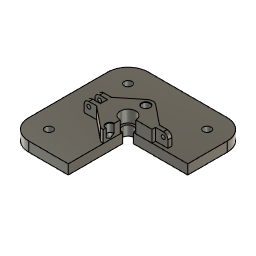
Sketch29_Final v2 (Autodesk Fusion 360 design; units mm, degrees)
Autodesk Fusion 360 part; units mm, degrees
sketch "Sketch2" plane through (0, 0, 0) normal (0, 0, 1) x (1, 0, 0)
  line L0 (102.0126, -154) -> (-102.0126, -154)
  line L1 (-154, -102.0126) -> (-154, 102.0126)
  line L2 (-102.0126, 154) -> (102.0126, 154)
  line L3 (154, 102.0126) -> (154, -102.0126)
  line L4 (138.7696, -138.7696) -> (-138.7696, 138.7696) construction
  line L5 (-138.7696, -138.7696) -> (138.7696, 138.7696) construction
  line L6 (0, 154) -> (-102, 154)
  line L7 (-154, 0) -> (-154, 102)
  circle A0 centre (-102, 102) radius 10
  circle A1 centre (102, 102) radius 10
  line L8 (-154, 0) -> (154, 0)
  circle A2 centre (-102, -102) radius 10
  circle A3 centre (102, -102) radius 10
  arc A4 (-101.9874, 154) -> (-154, 101.9874) centre (-102, 102) ccw
  arc A5 (154, 101.9874) -> (101.9874, 154) centre (102, 102) ccw
  arc A6 (101.9874, -154) -> (154, -101.9874) centre (102, -102) ccw
  arc A7 (-154, -101.9874) -> (-101.9874, -154) centre (-102, -102) ccw
  circle A8 centre (0, 0) radius 14
  dimension "d3" = 102
  dimension "d4" = 102
  dimension "d5" = 20
  dimension "d7" = 104
  dimension "d8" = 28
  constraint horizontal L0
  constraint perpendicular L0 L1
  constraint parallel L0 L2
  constraint parallel L1 L3
  constraint coincident L4 A8.centre
  constraint coincident L5 A8.centre
  constraint coincident A8.centre origin
  constraint parallel L2 L6
  constraint parallel L1 L7
  constraint coincident L4 A0.centre
  constraint concentric A0 A4
  constraint coincident L1.end A4
  constraint coincident L1 L7.start
  constraint coincident L2.start A4
  constraint coincident L2 L6.start
  constraint perpendicular L3 L8
  constraint symmetric A0 L8 A2
  constraint symmetric L8 A4 A7
  constraint symmetric L8 A5 A6
  constraint symmetric A1 L8 A3
  constraint coincident L2.end A5
  constraint coincident L3.start A5
  constraint coincident L3 L8.end
  constraint coincident L5.end A5
  constraint coincident L4.start A6
  constraint coincident L3.end A6
  constraint coincident L0.start A6
  constraint coincident L0.end A7
  constraint coincident L1.start A7
  constraint coincident L5.start A7
  constraint coincident L4.end A4
  constraint coincident L1 A4.end
  constraint coincident L2 A4.start
  constraint coincident L2 A5.end
  constraint coincident L3 A5.start
  constraint coincident L3 A6.end
  constraint coincident L0 A6.start
  constraint coincident L0 A7.end
  constraint coincident L1 A7.start
  measures "d3" distance of L6.start L6.end
  measures "d4" distance of L7.start L7.end
  measures "d5" diameter of A0
  measures "d7" diameter of A4
  measures "d8" diameter of A8
extrude "Extrude1" add sketch "Sketch2" along normal blind 25 contours L0 L1 L3 L8 A6 A7 A8 | L1 L2 L3 L6 L7 L8 A4 A5 A8 makes body 1
ref_plane "WorkPlane2" through (0, 77, 25) normal (0, 0, 1) x (1, 0, 0)
sketch "Sketch5" plane through (0, 77, 25) normal (0, 0, 1) x (1, 0, 0)
  circle A0 centre (0, -77) radius 20
  line L0 (0, -77) -> (20, -77)
  line L1 (0, -77) -> (0, -57)
  line L2 (0, -77) -> (62, -77)
  line L3 (62, -77) -> (62, -86)
  line L4 (62, -86) -> (94, -86)
  line L5 (94, -86) -> (94, -96)
  line L6 (94, -96) -> (62, -96)
  line L7 (0, -77) -> (0, -49)
  line L8 (62, -68) -> (94, -68)
  line L9 (94, -58) -> (62, -58)
  line L10 (94, -68) -> (94, -58)
  line L11 (62, -77) -> (62, -68)
  line L12 (62, -58) -> (11.3203, -17.0053)
  arc A1 (11.3203, -17.0053) -> (-11.3203, -17.0053) centre (0, -31) ccw
  line L13 (-94, -58) -> (-62, -58)
  line L14 (-62, -68) -> (-94, -68)
  line L15 (-94, -68) -> (-94, -58)
  line L16 (-62, -77) -> (-62, -68)
  line L17 (-62, -77) -> (-62, -86)
  line L18 (-62, -86) -> (-94, -86)
  line L19 (-94, -86) -> (-94, -96)
  line L20 (-94, -96) -> (-62, -96)
  line L21 (-62, -58) -> (-11.3203, -17.0053)
  line L22 (-62, -96) -> (-11.3203, -136.9947)
  arc A2 (-11.3203, -136.9947) -> (11.3203, -136.9947) centre (0, -123) ccw
  line L23 (62, -96) -> (11.3203, -136.9947)
  line L24 (0, -58) -> (26, -58)
  dimension "d22" = 40
  dimension "d23" = 62
  dimension "d24" = 9
  dimension "d25" = 32
  dimension "d26" = 10
  dimension "d27" = 32
  dimension "d28" = 46
  dimension "d29" = 36
  dimension "d58" = 26
  constraint coincident A0.centre L0.start
  constraint coincident A0 L0.end
  constraint horizontal L0
  constraint coincident A0 L1.end
  constraint perpendicular L0 L1
  constraint perpendicular L1 L2
  constraint perpendicular L2 L3
  constraint perpendicular L3 L4
  constraint perpendicular L4 L5
  constraint perpendicular L5 L6
  constraint perpendicular L2 L7
  constraint symmetric L3.start L2 L11.start
  constraint symmetric L2 L3.end L8.start
  constraint symmetric L2 L4.end L8.end
  constraint symmetric L2 L5.end L9.start
  constraint symmetric L2 L6.end L9.end
  constraint tangent L12 A1
  constraint symmetric L2.end L7 L16.start
  constraint symmetric L3.end L7 L17.end
  constraint symmetric L4.end L7 L18.end
  constraint symmetric L5.end L7 L19.end
  constraint symmetric L6.end L7 L20.end
  constraint symmetric L7 L8.start L14.start
  constraint symmetric L7 L8.end L14.end
  constraint symmetric L7 L9.start L13.start
  constraint symmetric L7 L9.end L13.end
  constraint symmetric L7 L2.end L16.start
  constraint symmetric L7 L12.end A1.end
  constraint symmetric L2 L9.end L6.end
  constraint symmetric L2 L12.end A2.end
  constraint symmetric L2 A1 A2
  constraint symmetric L2 L13.end L20.end
  constraint symmetric L2 A1.end L22.end
  constraint coincident L1 L24.start
  constraint perpendicular L1 L24
  measures "d22" diameter of A0
  measures "d23" distance of A0.centre L2.end
  measures "d24" distance of L2.end L3.end
  measures "d25" distance of L3.end L4.end
  measures "d26" distance of L4.end L5.end
  measures "d27" distance of L5.end L6.end
  measures "d28" distance of A0.centre A1.centre
  measures "d29" diameter of A1
  measures "d58" distance of L24.start L24.end
extrude "Extrude2" add sketch "Sketch5" along normal blind 31 separate body makes body 2
fillet "Fillet1" radius 12 1 edges at (94, -14, 56) on bodies 2
fillet "Fillet2" radius 12 1 edges at (94, 14, 56) on bodies 2
fillet "Fillet3" radius 12 1 edges at (-94, -14, 56) on bodies 2
fillet "Fillet4" radius 12 1 edges at (-94, 14, 56) on bodies 2
hole "Hole1" at (0, -46, 56) direction (0, 0, -1) diameter 20 depth 22 tip angle 118 countersink diameter 22 countersink angle 90 bodies 2
mirror "Mirror1" about plane through (0, 0, 0) normal (0, 1, 0) of "Hole1"
hole "Hole2" at (-82, -19, 44) direction (0, 1, 0) diameter 10 depth 10 tip angle 118 bodies 2
mirror "Mirror2" about plane through (0, 0, 0) normal (1, 0, 0) of "Hole2"
mirror "Mirror3" about plane through (0, 0, 0) normal (0, 1, 0) of "Hole2", "Mirror2"
sketch "Sketch6" plane through (0, 0, 0) normal (0, 0, 1) x (1, 0, 0)
  line L0 (0, 0) -> (160, 0)
  line L1 (160, 0) -> (160, -170)
  line L2 (160, -170) -> (0, -170)
  line L3 (0, -170) -> (0, 0)
  constraint horizontal L0
  constraint vertical L1
  constraint horizontal L2
  constraint vertical L3
  constraint coincident L0.start L3.end
extrude "Extrude3" cut sketch "Sketch6" along normal blind 70 bodies 1 2
